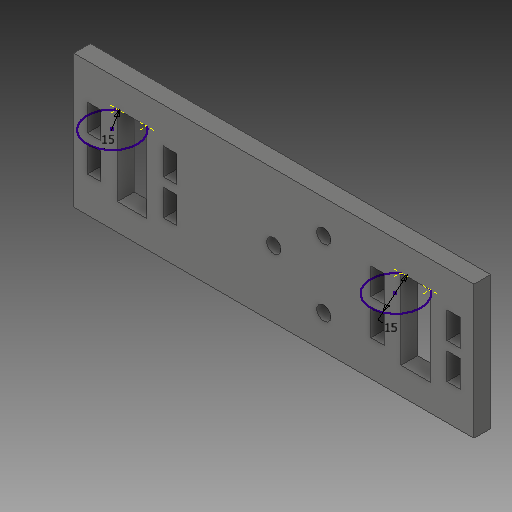
# Autodesk Inventor part: YCartFloor
Saved by Autodesk Inventor 2019 (Build 230136000, 136)
## iProperties
Created: 2019-08-21
Part Number: YCartFloor
Material: Generic
Document SubType Name: Modeling
Designer: Bruno
Density: 1 g/cm^3
Appearance: Default
Mass: 20.3952 g
Surface Area: 115.744 cm^2
Volume: 20.3952 cm^3
Author: Bruno
Autodesk Inventor part; units mm, degrees
ref_plane "YZ Plane" through (0, 0, 0) normal (1, 0, 0) x (0, 1, 0)
ref_plane "XZ Plane" through (0, 0, 0) normal (0, 1, 0) x (-1, 0, 0)
ref_plane "XY Plane" through (0, 0, 0) normal (0, 0, 1) x (1, 0, 0)
sketch "Sketch1" plane through (0, 0, 0) normal (0, 0, 1) x (1, 0, 0)
  line L0 (60, 0) -> (-60, 0)
  line L1 (-60, 0) -> (-60, -40)
  line L2 (-60, -40) -> (60, -40)
  line L3 (60, -40) -> (60, 0)
  line L4 (46.9, -8) -> (38.1, -8)
  line L5 (38.1, -8) -> (38.1, -32)
  line L6 (38.1, -32) -> (46.9, -32)
  line L7 (46.9, -32) -> (46.9, -8)
  line L8 (46.9, -8) -> (46.9, 0) construction
  line L9 (46.9, -32) -> (46.9, -40) construction
  line L10 (0, 0) -> (5.0949, 0) construction
  line L11 (-46.9, -8) -> (-38.1, -8)
  line L12 (-38.1, -8) -> (-38.1, -32)
  line L13 (-38.1, -32) -> (-46.9, -32)
  line L14 (-46.9, -32) -> (-46.9, -8)
  line L15 (-42.5, -23.6928) -> (-38.1, -23.6928) construction
  line L16 (-42.5, -23.6928) -> (-46.9, -23.6928) construction
  line L17 (46.9, -20) -> (60, -20) construction
  line L18 (-60, -20) -> (-46.9, -20) construction
  line L19 (51.9, -10.6667) -> (55.9, -10.6667)
  line L20 (55.9, -10.6667) -> (55.9, -18.6667)
  line L21 (55.9, -18.6667) -> (51.9, -18.6667)
  line L22 (51.9, -18.6667) -> (51.9, -10.6667)
  line L23 (51.9, -21.3333) -> (55.9, -21.3333)
  line L24 (55.9, -21.3333) -> (55.9, -29.3333)
  line L25 (55.9, -29.3333) -> (51.9, -29.3333)
  line L26 (51.9, -29.3333) -> (51.9, -21.3333)
  line L27 (51.9, -10.6667) -> (51.9, -8) construction
  line L28 (46.9, -8) -> (51.9, -8) construction
  line L29 (51.9, -18.6667) -> (51.9, -21.3333) construction
  line L30 (51.9, -29.3333) -> (51.9, -32) construction
  line L31 (46.9, -32) -> (51.9, -32) construction
  line L32 (29.1, -10.6667) -> (33.1, -10.6667)
  line L33 (33.1, -10.6667) -> (33.1, -18.6667)
  line L34 (33.1, -18.6667) -> (29.1, -18.6667)
  line L35 (29.1, -18.6667) -> (29.1, -10.6667)
  line L36 (29.1, -21.3333) -> (33.1, -21.3333)
  line L37 (33.1, -21.3333) -> (33.1, -29.3333)
  line L38 (33.1, -29.3333) -> (29.1, -29.3333)
  line L39 (29.1, -29.3333) -> (29.1, -21.3333)
  line L40 (38.1, -8) -> (33.1, -8) construction
  line L41 (33.1, -8) -> (33.1, -10.6667) construction
  line L42 (33.1, -18.6667) -> (33.1, -21.3333) construction
  line L43 (33.1, -29.3333) -> (33.1, -32) construction
  line L44 (33.1, -32) -> (38.1, -32) construction
  line L45 (-33.1, -10.6667) -> (-29.1, -10.6667)
  line L46 (-29.1, -10.6667) -> (-29.1, -18.6667)
  line L47 (-29.1, -18.6667) -> (-33.1, -18.6667)
  line L48 (-33.1, -18.6667) -> (-33.1, -10.6667)
  line L49 (-33.1, -21.3333) -> (-29.1, -21.3333)
  line L50 (-29.1, -21.3333) -> (-29.1, -29.3333)
  line L51 (-29.1, -29.3333) -> (-33.1, -29.3333)
  line L52 (-33.1, -29.3333) -> (-33.1, -21.3333)
  line L53 (-55.9, -29.3333) -> (-51.9, -29.3333)
  line L54 (-51.9, -29.3333) -> (-51.9, -21.3333)
  line L55 (-51.9, -21.3333) -> (-55.9, -21.3333)
  line L56 (-55.9, -21.3333) -> (-55.9, -29.3333)
  line L57 (-51.9, -10.6667) -> (-55.9, -10.6667)
  line L58 (-55.9, -10.6667) -> (-55.9, -18.6667)
  line L59 (-55.9, -18.6667) -> (-51.9, -18.6667)
  line L60 (-51.9, -18.6667) -> (-51.9, -10.6667)
  line L61 (-33.1, -29.3333) -> (-38.1, -29.3333) construction
  line L62 (-51.9, -29.3333) -> (-46.9, -29.3333) construction
  circle A0 centre (15, -30) radius 2.125
  circle A1 centre (15, -10) radius 2.125
  line L63 (15, -10) -> (15, -30) construction
  line L64 (15, -30) -> (15, -40) construction
  line L65 (15, -10) -> (15, 0) construction
  circle A2 centre (0, -20) radius 2.125
  line L66 (0, -20) -> (0, -40) construction
  line L67 (0, -20) -> (0, 0) construction
  dimension "d0" = 120
  dimension "d1" = 40
  dimension "d2" = 8.8
  dimension "d3" = 24
  dimension "d4" = 8.8
  dimension "d5" = 24
  dimension "d6" = 4
  dimension "d7" = 8
  dimension "d8" = 5
  dimension "d11" = 76.2
  dimension "d14" = 4.25
  dimension "d15" = 4.25
  dimension "d16" = 20
  dimension "d17" = 45
  dimension "d18" = 4.25
  constraints: 136 end point, 24 equal length, 22 parallel, 18 perpendicular, 18 point on line, 15 horizontal, 8 collinear, 6 vertical, 5 midpoint, 3 centre point
  measures "d0" distance of L1.end L2.end
  measures "d1" distance of L2.end L0.start
  measures "d2" distance of L6.end L5.end
  measures "d3" distance of L5.end L4.end
  measures "d4" distance of L12.end L13.end
  measures "d5" distance of L11.end L12.end
  measures "d6" distance of L20.end L21.end
  measures "d7" distance of L19.end L20.end
  measures "d8" distance between parallel lines of L7 L22
  measures "d11" distance between parallel lines of L12 L5
  measures "d14" diameter of A0
  measures "d15" diameter of A1
  measures "d16" distance of L63.start L63.end
  measures "d17" distance between parallel lines of L3 L63
  measures "d18" diameter of A2
extrude "Extrusion1" add sketch "Sketch1" along normal blind 5
sketch "Sketch2" plane through (-46.9, -8, 0) normal (0, -1, 0) x (1, 0, 0)
  circle A0 centre (4.4, 11.0737) radius 7.5
  circle A1 centre (89.4, 11.0737) radius 7.5
  point P0 (46.9, 0)
  point P1 (0, 5)
  point P2 (8.8, 5)
  point P3 (85, 5)
  point P4 (93.8, 5)
  dimension "d12" = 15
  dimension "d13" = 15
  constraints: 4 point on circle, 2 centre point
  measures "d12" diameter of A0
  measures "d13" diameter of A1
body "Solid1"
